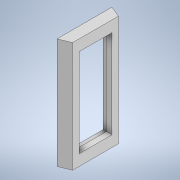
# Autodesk Inventor part: SatelliteSideWallSensor
Saved by Autodesk Inventor 2020 (Build 240168000, 168)
## iProperties
Created: 2020-02-24
Part Number: SatelliteSideWallSensor
Material: Generic
Document SubType Name: Modeling
Designer: WANG
Density: 1 g/cm^3
Appearance: Default
Author: WANG
Autodesk Inventor part; units mm, degrees
ref_plane "YZ Plane" through (0, 0, 0) normal (1, 0, 0) x (0, 1, 0)
ref_plane "XZ Plane" through (0, 0, 0) normal (0, 1, 0) x (-1, 0, 0)
ref_plane "XY Plane" through (0, 0, 0) normal (0, 0, 1) x (1, 0, 0)
sketch "Sketch1" plane through (0, 0, 0) normal (0, 1, 0) x (-1, 0, 0)
  line L0 (0, 0) -> (152.4, 0) construction
  line L1 (152.4, 0) -> (152.4, -152.4) construction
  line L2 (152.4, -152.4) -> (0, -152.4) construction
  line L3 (0, -152.4) -> (0, 0) construction
  line L4 (44.6369, -152.4) -> (0, -107.7631) construction
  line L5 (0, -107.7631) -> (0, -44.6369) construction
  line L6 (0, -44.6369) -> (44.6369, 0) construction
  line L7 (44.6369, 0) -> (107.7631, 0) construction
  line L8 (107.7631, 0) -> (152.4, -44.6369) construction
  line L9 (152.4, -44.6369) -> (152.4, -107.7631) construction
  line L10 (152.4, -107.7631) -> (107.7631, -152.4) construction
  line L11 (107.7631, -152.4) -> (44.6369, -152.4) construction
  line L12 (102.5026, -12.7) -> (139.7, -49.8974) construction
  line L13 (139.7, -49.8974) -> (139.7, -102.5026) construction
  line L14 (139.7, -102.5026) -> (102.5026, -139.7) construction
  line L15 (102.5026, -139.7) -> (49.8974, -139.7) construction
  line L16 (49.8974, -139.7) -> (12.7, -102.5026) construction
  line L17 (12.7, -102.5026) -> (12.7, -49.8974) construction
  line L18 (12.7, -49.8974) -> (49.8974, -12.7) construction
  line L19 (49.8974, -12.7) -> (102.5026, -12.7) construction
  line L20 (152.4, -44.6369) -> (139.7, -49.8974)
  line L21 (139.7, -49.8974) -> (139.7, -102.5026)
  line L22 (152.4, -107.7631) -> (139.7, -102.5026)
  line L23 (152.4, -107.7631) -> (152.4, -44.6369)
  point P0 (76.2, -76.2)
  point P1 (76.2, -76.2)
  point P2 (76.2, -76.2)
  dimension "d0" = 152.4
  dimension "d1" = 152.4
  dimension "d2" = 12.7
  dimension "d3" = 63.1262
  dimension "d4" = 52.6051
  constraints: 48 end point, 5 collinear, 2 coincident, 2 horizontal, 2 parallel, 1 perpendicular, 1 point on line, 34 other
  measures "d0" distance of L2.start L2.end
  measures "d1" distance of L1.start L2.start
  measures "d2" distance between parallel lines of L13 L9
  measures "d3" distance of L10.start L11.start
  measures "d4" distance of L14.start L15.start
extrude "Extrusion1" add sketch "Sketch1" along normal blind 127
sketch "Sketch2" plane through (-152.4, 0, -107.7631) normal (-1, 0, 0) x (0, 0, 1)
  line L0 (63.1261, 0) -> (63.1261, 127) projected
  line L1 (0, 127) -> (63.1261, 127) projected
  line L2 (0, 0) -> (0, 127) projected
  line L3 (0, 0) -> (63.1261, 0) projected
  line L4 (12.7, 114.3) -> (50.4261, 114.3)
  line L5 (50.4261, 114.3) -> (50.4261, 12.7)
  line L6 (50.4261, 12.7) -> (12.7, 12.7)
  line L7 (12.7, 12.7) -> (12.7, 114.3)
  point P0 (107.7631, 0)
  point P1 (12.7, 12.7)
  dimension "d7" = 12.7
  dimension "d8" = 12.7
  dimension "d9" = 12.7
  dimension "d10" = 12.7
  dimension "d11" = 12.7
  dimension "d12" = 12.7
  dimension "d13" = 12.7
  dimension "d14" = 12.7
  constraints: 8 end point, 2 parallel, 1 horizontal, 1 perpendicular
  measures "d7" distance from line of L0 point (50.426, 114.3)
  measures "d8" distance from line of L1 point (50.426, 114.3)
  measures "d9" distance from line of L2 L4.start
  measures "d10" distance from line of L1 L4.start
  measures "d11" distance from line of point (12.7, 12.7) L2
  measures "d12" distance from line of L3 point (12.7, 12.7)
  measures "d13" distance from line of L3 L5.end
  measures "d14" distance from line of L0 L5.end
extrude "Extrusion2" cut sketch "Sketch2" against normal up to surface (12.7 mm away) contours L4 L5 L6 L7
sketch "Sketch4" plane through (-152.4, 0, -107.7631) normal (-1, 0, 0) x (0, 0, 1)
  line L0 (0, 127) -> (63.1261, 127) projected
  line L1 (0, 0) -> (0, 127) projected
  line L2 (0, 0) -> (63.1261, 0) projected
  line L3 (63.1261, 0) -> (63.1261, 127) projected
  line L4 (10.16, 116.84) -> (52.9661, 116.84)
  line L5 (52.9661, 116.84) -> (52.9661, 10.16)
  line L6 (52.9661, 10.16) -> (10.16, 10.16)
  line L7 (10.16, 10.16) -> (10.16, 116.84)
  line L8 (50.4261, 114.3) -> (12.7, 114.3) projected
  line L9 (50.4261, 114.3) -> (50.4261, 12.7) projected
  line L10 (12.7, 114.3) -> (50.4261, 114.3)
  line L11 (50.4261, 114.3) -> (50.4261, 12.7)
  line L12 (50.4261, 12.7) -> (12.7, 12.7)
  line L13 (12.7, 12.7) -> (12.7, 114.3)
  point P0 (107.7631, 0)
  dimension "d17" = 10.16
  dimension "d18" = 10.16
  dimension "d19" = 10.16
  dimension "d20" = 10.16
  constraints: 16 end point, 4 parallel, 2 horizontal, 2 perpendicular
  measures "d17" distance from line of L4.start L0
  measures "d18" distance from line of L1 L4.start
  measures "d19" distance from line of L2 L5.end
  measures "d20" distance from line of L3 L5.end
extrude "Extrusion3" cut sketch "Sketch4" against normal blind 6.35 contours L4 L5 L6 L7
equation "\"d9\" = d8"
equation "\"d10\" = d8"
equation "\"d11\" = d9"
equation "\"d12\" = d9"
equation "\"d13\" = d9"
equation "\"d14\" = d9"
body "Solid1"
